Pinion Gear Bearing insert_v1 (Autodesk Fusion 360 design; units mm, degrees)
Autodesk Fusion 360 part; units mm, degrees
note: some values were not read from the file. Set by a fixed rule: which sketch regions a step uses.
sketch "Sketch2" plane through (0, 0, 0) normal (0, 1, 0) x (1, 0, 0)
  line L0 (0, 0) -> (0, -3.5) construction
  line L1 (0, -3.5) -> (8.2, -3.5) construction
  circle A0 centre (8.2, -3.5) radius 3
  line L2 (5.2, -3.5) -> (11.2, -3.5)
  line L3 (11.2, 1) -> (5.2, 1)
  line L4 (5.2, 1) -> (5.2, -2)
  line L5 (5.2, -2) -> (11.2, -2)
  line L6 (11.2, -2) -> (11.2, 1)
  line L7 (11.2, 1) -> (5.2, -2) construction
  line L8 (5.2, 1) -> (11.2, -2) construction
  point P0 (8.2, -0.5)
  dimension "d1" = 3.5
  dimension "d2" = 8.2
  dimension "d3" = 6
  dimension "d4" = 6
  dimension "d10" = 6
  dimension "d11" = 3
  dimension "d12" = 1.5
  constraint coincident L0.start origin
  constraint vertical L0
  constraint perpendicular L0 L1
  constraint coincident L1.end A0.centre
  constraint horizontal L2
  constraint coincident L1 L2.start
  constraint coincident A0 L2.start
  constraint horizontal L3
  constraint perpendicular L3 L4
  constraint parallel L3 L5
  constraint parallel L4 L6
  constraint coincident L7 P0
  constraint coincident L8 P0
  measures "d1" distance of L0.start L0.end
  measures "d2" distance of L0.end L1.end
  measures "d3" diameter of A0
  measures "d4" distance of L2.start L2.end
  measures "d10" distance of L4.end L5.end
  measures "d11" distance of L3.end L4.end
  measures "d12" distance of L1.end L5
revolve "Revolve1" add sketch "Sketch2" angle 360 about axis through (0, 0, 0) along (0, 0, 1) contours A0 L3 L4 L5 L6
